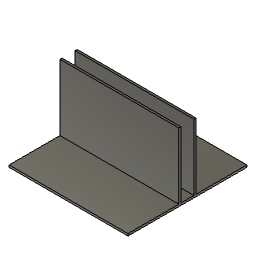
Laptop Vertical Holder Temporary v4 (Autodesk Fusion 360 design; units mm, degrees)
Autodesk Fusion 360 part; units mm, degrees
sketch "Sketch1" plane through (0, 0, 0) normal (0, 0, 1) x (1, 0, 0)
  line L0 (114.3, 114.3) -> (-114.3, 114.3)
  line L1 (-114.3, 114.3) -> (-114.3, -114.3)
  line L2 (-114.3, -114.3) -> (114.3, -114.3)
  line L3 (114.3, -114.3) -> (114.3, 114.3)
  line L4 (114.3, 114.3) -> (-114.3, -114.3) construction
  line L5 (-114.3, 114.3) -> (114.3, -114.3) construction
  line L6 (0, 0) -> (114.3, 0)
  line L7 (0, 0) -> (-114.3, 0)
  line L8 (-114.3, 0) -> (-114.3, 12.5)
  line L9 (-114.3, 12.5) -> (114.3, 12.5)
  line L10 (-114.3, -12.5) -> (114.3, -12.5)
  line L11 (-114.3, -16.5) -> (114.3, -16.5)
  line L12 (-114.3, 16.5) -> (114.3, 16.5)
  dimension "d1" = 228.6
  dimension "d2" = 228.6
  dimension "d3" = 12.5
  dimension "d4" = 4
  constraint horizontal L0
  constraint perpendicular L0 L1
  constraint parallel L0 L2
  constraint parallel L1 L3
  constraint coincident L4 L6.start
  constraint coincident L5 L6.start
  constraint coincident L6.start L7.start
  constraint midpoint L3 L6.end
  constraint midpoint L1 L7.end
  constraint perpendicular L7 L8
  constraint coincident L3 L9.end
  constraint perpendicular L3 L9
  constraint symmetric L6 L8.end L10.start
  constraint symmetric L6 L9.end L10.end
  constraint symmetric L6 L11.start L12.start
  constraint symmetric L6 L11.end L12.end
  measures "d1" distance of L1.end L2.end
  measures "d2" distance of L0.end L1.end
  measures "d3" distance of L7.end L8.end
extrude "Extrude1" add sketch "Sketch1" against normal blind 4
extrude "Extrude2" add sketch "Sketch1" along normal blind 127 contours L1 L3 L9 L12 | L1 L3 L10 L11
